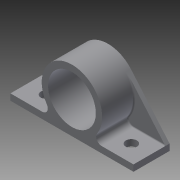
# Autodesk Inventor part: northrop bearing housing thru .5b
Saved by Autodesk Inventor 2015 (Build 190159000, 159)
## iProperties
Created: 2014-02-03
Part Number: northrop bearing housing thru .5b
Material: Generic
Document SubType Name: Modeling
Designer: CakeSpy
Density: 1 g/cm^3
Appearance: Default
Author: CakeSpy
Autodesk Inventor part; units mm, degrees
ref_plane "YZ Plane" through (0, 0, 0) normal (1, 0, 0) x (0, 1, 0)
ref_plane "XZ Plane" through (0, 0, 0) normal (0, 1, 0) x (-1, 0, 0)
ref_plane "XY Plane" through (0, 0, 0) normal (0, 0, 1) x (1, 0, 0)
sketch "Sketch1" plane through (0, 0, 0) normal (0, 0, 1) x (1, 0, 0)
  line L0 (0, 50.292) -> (0, -8.382)
  line L1 (-67.564, 0) -> (67.564, 0)
  circle A0 centre (0, 19.05) radius 14.2875
  line L2 (-36.83, 0) -> (-36.83, 3.81)
  arc A1 (15.019707, 8.954065) -> (-15.019707, 8.954065) centre (0, 19.05) ccw
  line L3 (-36.83, 3.81) -> (-13.757917, 30.807518)
  line L4 (-36.83, 0) -> (36.83, 0)
  line L5 (36.83, 3.81) -> (13.757917, 30.807518)
  line L6 (36.83, 0) -> (36.83, 3.81)
  line L7 (-36.83, 3.81) -> (-17.760145, 3.81)
  line L8 (36.83, 3.81) -> (17.760145, 3.81)
  arc A2 (-17.760145, 3.81) -> (-15.019707, 8.954065) centre (-17.760145, 7.112) ccw
  arc A3 (15.019707, 8.954065) -> (17.760145, 3.81) centre (17.760145, 7.112) ccw
  circle A4 centre (0, 19.05) radius 10.795
  circle A5 centre (0, 19.05) radius 6.35 construction
  point P0 (0, 0)
  point P1 (9.760221, 3.81)
  point P2 (-9.760221, 3.81)
  dimension "d0" = 28.575
  dimension "d1" = 3.81
  dimension "d2" = 19.05
  dimension "d3" = 36.83
  dimension "d4" = 36.83
  dimension "d5" = 3.302
  dimension "d6" = 3.302
  dimension "d7" = 3.81
  dimension "d8" = 3.81
  dimension "d17" = 21.59
  dimension "d18" = 12.7
  constraints: 14 end point, 10 point on circle, 6 centre point, 6 tangent, 5 point on line, 3 coincident, 3 perpendicular, 1 collinear
  measures "d0" diameter of A0
  measures "d1" radial gap between concentric circles of A1 A0
  measures "d2" distance from line of A0.centre L1
  measures "d3" distance between parallel lines of L6 L0
  measures "d4" distance between parallel lines of L2 L0
  measures "d5" radius of A2
  measures "d6" radius of A3
  measures "d7" distance of L4.end L5.start
  measures "d8" distance of L2.start L2.end
  measures "d17" diameter of A4
  measures "d18" diameter of A5
sketch "Sketch3" plane through (0, 0, 0) normal (0, 1, 0) x (-1, 0, 0)
  line L0 (-67.564, 0) -> (67.564, 0) projected
  circle A0 centre (-25.4, 11.43) radius 3.302
  line L1 (0, 5.4356) -> (0, 24.2824) projected
  circle A1 centre (25.4, 11.43) radius 3.302
  dimension "d23" = 11.43
  dimension "d24" = 25.4
  dimension "d25" = 6.604
  constraints: 2 centre point, 1 symmetric about line, 1 other
  measures "d23" distance from line of A0.centre L0
  measures "d24" distance from line of A0.centre L1
  measures "d25" diameter of A0
extrude "Extrusion3" add sketch "Sketch1" along normal blind 21.59 contours A1 A3 L8 L6 L1 L0 A0 | L0 A0 L1 L2 L7 A2 A1
extrude "Extrusion4" add sketch "Sketch1" along normal blind 2.54 contours A1 A3 L8 L6 L1 L0 A0 | L0 A0 L1 L2 L7 A2 A1 | L5 L8 A3 A1 | A1 A2 L7 L3
extrude "Extrusion5" cut sketch "Sketch3" along normal through all
fillet "Fillet1" radius 0.762 3 edges at (14.8459, 5.5595, 2.54) (18.0674, 20.0932, 2.54) (27.2951, 3.81, 2.54)
fillet "Fillet2" radius 0.762 3 edges at (-27.2951, 3.81, 2.54) (-14.8459, 5.5595, 2.54) (-18.0674, 20.0932, 2.54)
sketch "Sketch4" plane through (0, 0, 21.59) normal (0, 0, 1) x (1, 0, 0)
  circle A0 centre (0, 19.05) radius 14.2875
  line L0 (36.83, 0) -> (36.83, 3.81)
  line L1 (36.83, 3.81) -> (17.760145, 3.81)
  arc A1 (15.019707, 8.954065) -> (17.760145, 3.81) centre (17.760145, 7.112) ccw
  arc A2 (15.019707, 8.954065) -> (-15.019707, 8.954065) centre (0, 19.05) ccw
  arc A3 (-17.760145, 3.81) -> (-15.019707, 8.954065) centre (-17.760145, 7.112) ccw
  line L2 (-17.760145, 3.81) -> (-36.83, 3.81)
  line L3 (-36.83, 3.81) -> (-36.83, 0)
  line L4 (-36.83, 0) -> (36.83, 0)
  line L5 (-49.53, 41.91) -> (49.53, 41.91)
  line L6 (49.53, 41.91) -> (49.53, 3.81)
  line L7 (49.53, 3.81) -> (-49.53, 3.81)
  line L8 (-49.53, 3.81) -> (-49.53, 41.91)
  point P0 (0, 0)
  dimension "d30" = 0
  dimension "d31" = 38.1
  dimension "d32" = 12.7
  dimension "d33" = 12.7
  constraints: 8 end point, 2 parallel, 1 horizontal, 1 perpendicular
  measures "d30" distance between parallel lines of L7 L2
  measures "d31" distance of L7.end L5.start
  measures "d32" distance between parallel lines of L6 L0
  measures "d33" distance between parallel lines of L8 L3
equation "\"d3\" = d4"
equation "\"d6\" = d5"
equation "\"d8\" = d7"
body "Solid2"
